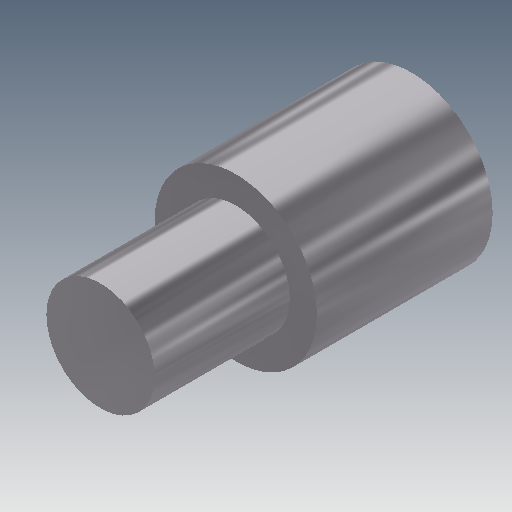
# Autodesk Inventor part: WeldExer_lower_sleeve
Saved by Autodesk Inventor 2020.1 (Build 241239000, 239)
## iProperties
Part Number: WeldExer_lower_sleeve
Document SubType Name: Modeling
Created: 2003-07-06
Designer: Ronald Myers
Manufacturer: Standard
Standards Organization: Custom
Stock Number: WeldExer_lower_sleeve
Density: 1 g/cm^3
Material: Generic
Appearance: Aluminum (Polished)
Control State: 0
Master: False
Checked Out: False
Shininess: 64.0
Length Units: 11269
Angle Units: 11279
Time Units: 11290
Mass Units: 11286
Length Display Precision: 3
Angle Display Precision: 2
Compacted: True
Density: 0.0
Volumn: 0.0
Area: 0.0
PropertySet Name: Model Information
Author: Ronald Myers
Autodesk Inventor part; units mm, degrees
ref_plane "YZ Plane" through (0, 0, 0) normal (1, 0, 0) x (0, 1, 0)
ref_plane "XZ Plane" through (0, 0, 0) normal (0, 1, 0) x (-1, 0, 0)
ref_plane "XY Plane" through (0, 0, 0) normal (0, 0, 1) x (1, 0, 0)
sketch "Sketch1" plane through (0, 0, 0) normal (0, 0, 1) x (1, 0, 0)
  circle A0 centre (-2.6525, -0.9947) radius 6
  dimension "d0" = 12
  constraints: 1 centre point
  measures "d0" diameter of A0
extrude "Extrusion1" add sketch "Sketch1" along normal blind 23
sketch "Sketch2" plane through (-2.6525, -0.9947, 23) normal (0, 0, 1) x (1, 0, 0)
  circle A0 centre (0, 0) radius 6 projected
  circle A1 centre (0, 0) radius 4
  dimension "d3" = 8
  constraints: 1 centre point, 1 coincident
  measures "d3" diameter of A1
extrude "Extrusion2" cut sketch "Sketch2" against normal blind 10
body "Solid1"
